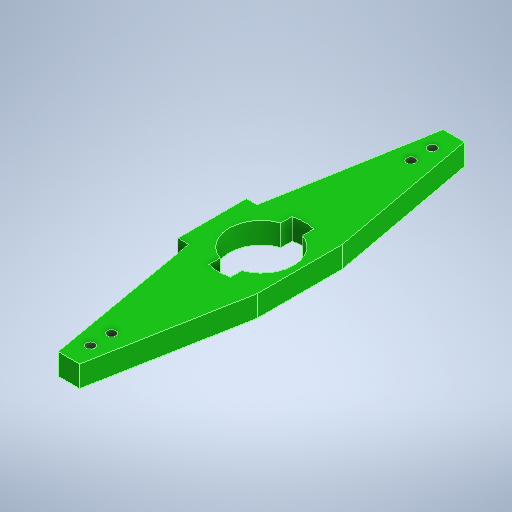
# Autodesk Inventor part: Axe centrale
Saved by Autodesk Inventor 2025.2 (Build 292293000, 293)
## iProperties
Created: 2026-03-16
Part Number: Axe centrale
Material: Générique
Document SubType Name: Modeling
Designer: genon
Density: 1 g/cm^3
Appearance: Vert foncé
Author: genon
Autodesk Inventor part; units mm, degrees
ref_plane "YZ Plane" through (0, 0, 0) normal (1, 0, 0) x (0, 1, 0)
ref_plane "XZ Plane" through (0, 0, 0) normal (0, 1, 0) x (-1, 0, 0)
ref_plane "XY Plane" through (0, 0, 0) normal (0, 0, 1) x (1, 0, 0)
sketch "Esquisse1" plane through (0, 0, 0) normal (0, 1, 0) x (-1, 0, 0)
  circle A0 centre (0, 0) radius 15.1
  line L0 (0, 0) -> (18, 0)
  line L1 (18, 0) -> (18, -16)
  line L2 (18, 0) -> (18, 16)
  line L3 (18, 16) -> (23, 16)
  line L4 (23, 16) -> (23, -16)
  line L5 (23, -16) -> (18, -16)
  line L6 (0, 0) -> (-18, 0)
  line L7 (-18, 0) -> (-18, -20)
  line L8 (-18, 0) -> (-18, 20)
  line L9 (0, 0) -> (0, 90)
  line L10 (0, 0) -> (90, 0) construction
  line L11 (0, 90) -> (-5, 90)
  line L12 (-5, 90) -> (-18, 20)
  line L13 (0, 90) -> (5, 90)
  line L14 (5, 90) -> (18, 16)
  line L15 (0, 0) -> (0, -90)
  line L16 (0, 0) -> (90, 0) construction
  line L17 (0, -90) -> (5, -90)
  line L18 (5, -90) -> (18, -16)
  line L19 (0, -90) -> (-5, -90)
  line L20 (-5, -90) -> (-18, -20)
  line L21 (0, 0) -> (5.1, 0)
  line L22 (5.1, 0) -> (5.1, -19.4422)
  line L23 (0, 0) -> (-5.1, 0)
  line L24 (-5.1, 0) -> (-5.1, -19.4422)
  line L25 (-5.1, 0) -> (-5.1, 19.4422)
  line L26 (5.1, 0) -> (5.1, 19.4422)
  arc A1 (-5.1, -19.4422) -> (5.1, -19.4422) centre (0, 0) ccw
  arc A2 (5.1, 19.4422) -> (-5.1, 19.4422) centre (0, 0) ccw
  point P0 (5.1, -14.2127)
  point P1 (-5.1, -14.2127)
  point P2 (-5.1, 14.2127)
  point P3 (5.1, 14.2127)
  dimension "d0" = 30.2
  dimension "d1" = 18
  dimension "d2" = 16
  dimension "d3" = 90
  dimension "d4" = 16
  dimension "d5" = 5
  dimension "d6" = 18
  dimension "d7" = 20
  dimension "d8" = 20
  dimension "d9" = 90
  dimension "d10" = 90
  dimension "d11" = 5
  dimension "d12" = 5
  dimension "d13" = 90
  dimension "d14" = 90
  dimension "d15" = 5
  dimension "d16" = 90
  dimension "d17" = 5
  dimension "d19" = 5.1
  dimension "d20" = 5.1
  constraints: 54 end point, 12 perpendicular, 5 horizontal, 5 point on line, 4 point on circle, 3 centre point, 3 vertical, 2 coincident
  measures "d0" diameter of A0
  measures "d1" distance of L0.start L0.end
  measures "d2" distance of L0.end L1.end
  measures "d3" angle of L0 L1
  measures "d4" distance of L0.end L2.end
  measures "d5" distance of L2.end L3.end
  measures "d6" distance of L0.start L6.end
  measures "d7" distance of L6.end L7.end
  measures "d8" distance of L6.end L8.end
  measures "d9" distance of L0.start L9.end
  measures "d10" angle of L10 L9
  measures "d11" distance of L9.end L11.end
  measures "d12" distance of L9.end L13.end
  measures "d13" distance of L0.start L15.end
  measures "d14" angle of L15 L16
  measures "d15" distance of L15.end L17.end
  measures "d16" angle of L17 L15
  measures "d17" distance of L15.end L19.end
  measures "d19" distance of L21.start L21.end
  measures "d20" distance of L21.start L23.end
extrude "Extrusion1" add sketch "Esquisse1" along normal blind 10 contours L0 L1 L18 L17 L15 A1 L22 A0 | A0 L26 A2 L9 L13 L14 L2 L0 | L2 L3 L4 L5 L1 | A0 L6 L8 L12 L11 L9 A2 L25 | L24 A1 L15 L19 L20 L7 L6 A0
sketch "Esquisse2" plane through (0, 10, 0) normal (0, 1, 0) x (1, 0, 0)
  line L0 (-5, -90) -> (5, -90) projected
  line L1 (0, -90) -> (0, -60)
  line L2 (0, -60) -> (-10.2703, -60)
  line L3 (-18, -16) -> (-5, -90) projected
  line L4 (0, -60) -> (10.5714, -60)
  line L5 (5, -90) -> (18, -20) projected
  line L6 (0, -90) -> (0, -80)
  line L7 (0, -80) -> (0, -70)
  line L8 (0, 0) -> (-7.091, 0)
  point P0 (0, 80)
  point P1 (0, 70)
  dimension "d23" = 30
  dimension "d24" = 10
  dimension "d25" = 10
  constraints: 12 end point, 4 point on line, 2 coincident, 2 horizontal, 2 symmetric about line, 1 midpoint, 1 perpendicular, 1 vertical
  measures "d23" distance of L1.start L1.end
  measures "d24" distance of L1.start L6.end
  measures "d25" distance of L6.end L7.end
hole "Perçage1" at (0, 10, 80) at (0, 10, 70) at (0, 10, -70) at (0, 10, -80) direction (0, -1, 0) diameter 4.134 end through all thread size "M5x0.8" class "6H" standard "ISO Metric profile"
